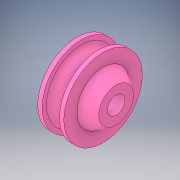
# Autodesk Inventor part: line pulley
Saved by Autodesk Inventor 2017 SP1 (Build 210196100, 196)
## iProperties
Created: 2018-01-29
Part Number: line pulley
Material: ABS Plastic
Document SubType Name: Modeling
Designer: Ben
Density: 1.06 g/cm^3
Appearance: Pink
Author: Ben
Autodesk Inventor part; units mm, degrees
ref_plane "YZ Plane" through (0, 0, 0) normal (1, 0, 0) x (0, 1, 0)
ref_plane "XZ Plane" through (0, 0, 0) normal (0, 1, 0) x (-1, 0, 0)
ref_plane "XY Plane" through (0, 0, 0) normal (0, 0, 1) x (1, 0, 0)
sketch "Sketch1" plane through (0, 0, 0) normal (0, 0, 1) x (1, 0, 0)
  arc A0 (-3.175, 12.7) -> (3.175, 12.7) centre (0, 12.7) ccw
  line L0 (0, -1.6305) -> (0, 0) construction
  line L1 (0, -1.6305) -> (0, 9.525) construction
  line L2 (3.175, 12.7) -> (3.175, 14.2875)
  line L3 (3.175, 14.2875) -> (4.7625, 14.2875)
  line L4 (4.7625, 14.2875) -> (4.7625, 9.525)
  line L5 (-3.175, 12.7) -> (-3.175, 14.2875)
  line L6 (-3.175, 14.2875) -> (-4.7625, 14.2875)
  line L7 (-4.7625, 14.2875) -> (-4.7625, 9.525)
  line L8 (9.525, 3.175) -> (-9.525, 3.175)
  line L9 (3.175, 12.7) -> (-3.175, 12.7) construction
  line L10 (9.525, 6.35) -> (9.525, 3.175)
  line L11 (-9.525, 6.35) -> (-9.525, 3.175)
  line L12 (9.525, 6.35) -> (4.7625, 9.525)
  line L13 (-4.7625, 9.525) -> (-9.525, 6.35)
  line L14 (21.4144, 0) -> (-14.6121, 0) construction
  point P0 (0, 3.175)
  dimension "d1" = 1.5875
  dimension "d2" = 1.5875
  dimension "d7" = 9.525
  dimension "d8" = 3.175
  dimension "d10" = 3.175
  dimension "d11" = 9.525
  dimension "d12" = 19.05
  dimension "d13" = 3.175
  dimension "d14" = 3.175
  constraints: 30 end point, 6 perpendicular, 4 equal length, 3 horizontal, 3 point on circle, 3 point on line, 3 vertical, 1 centre point, 1 collinear, 1 midpoint
  measures "d1" distance of L2.start L2.end
  measures "d2" distance of L2.end L3.end
  measures "d7" distance of L0.end L1.end
  measures "d8" distance from line of L0.end L8
  measures "d10" distance from line of L1.end L9
  measures "d11" distance between parallel lines of L7 L4
  measures "d12" distance of L8.start L8.end
  measures "d13" distance of L10.start L8.start
  measures "d14" vertical distance of L10.start L4.end
revolve "Revolution1" add sketch "Sketch1" angle 360 about axis through (21.4144, 0, 0) along (-1, 0, 0)
body "Solid1"
